Autodesk Fusion 360 part; units mm, degrees
(part 3 of 11)
  spline S34 degree 5 poles (-69.3976, -46.666) (-69.4262, -46.6856) (-69.4827, -46.7255) (-69.566, -46.7874) (-69.6741, -46.8736) (-69.8053, -46.9865) (-69.9336, -47.103) (-70.0602, -47.2219) (-70.1858, -47.342) (-70.3108, -47.4628) (-70.435, -47.5846) (-70.5583, -47.7074) (-70.6804, -47.8317) (-70.801, -47.9578) (-70.9202, -48.0856) (-71.038, -48.215) (-71.1547, -48.3457) (-71.2704, -48.4776) (-71.3852, -48.6104) (-71.4992, -48.7441) (-71.6124, -48.8787) (-71.7247, -49.0142) (-71.8361, -49.1508) (-71.9465, -49.2883) (-72.0561, -49.4269) (-72.1647, -49.5664) (-72.2724, -49.7069) (-72.3794, -49.8482) (-72.4855, -49.9903) (-72.5909, -50.1332) (-72.6954, -50.2769) (-72.7992, -50.4214) (-72.9023, -50.5667) (-73.0045, -50.7127) (-73.106, -50.8595) (-73.2067, -51.0071) (-73.3066, -51.1554) (-73.4058, -51.3044) (-73.5043, -51.4541) (-73.6021, -51.6045) (-73.6991, -51.7555) (-73.7954, -51.9073) (-73.8911, -52.0596) (-73.986, -52.2127) (-74.0802, -52.3664) (-74.1737, -52.5207) (-74.2665, -52.6757) (-74.3586, -52.8312) (-74.45, -52.9874) (-74.5408, -53.1442) (-74.6309, -53.3016) (-74.7203, -53.4595) (-74.8091, -53.618) (-74.8972, -53.7772) (-74.9846, -53.9368) (-75.0713, -54.097) (-75.1575, -54.2578) (-75.2429, -54.4191) (-75.3277, -54.581) (-75.4119, -54.7434) (-75.4954, -54.9063) (-75.5783, -55.0698) (-75.6605, -55.2337) (-75.7421, -55.3982) (-75.8231, -55.5632) (-75.9034, -55.7287) (-75.9831, -55.8946) (-76.0622, -56.0611) (-76.1407, -56.228) (-76.2185, -56.3954) (-76.2957, -56.5633) (-76.357, -56.698) (-76.4027, -56.7993) (-76.433, -56.8669) (-76.4482, -56.9007) knots 0 0 0 0 0 0 0.01428571 0.02857143 0.04285714 0.05714286 0.07142857 0.08571429 0.1 0.11428571 0.12857143 0.14285714 0.15714286 0.17142857 0.18571429 0.2 0.21428571 0.22857143 0.24285714 0.25714286 0.27142857 0.28571429 0.3 0.31428571 0.32857143 0.34285714 0.35714286 0.37142857 0.38571429 0.4 0.41428571 0.42857143 0.44285714 0.45714286 0.47142857 0.48571429 0.5 0.51428571 0.52857143 0.54285714 0.55714286 0.57142857 0.58571429 0.6 0.61428571 0.62857143 0.64285714 0.65714286 0.67142857 0.68571429 0.7 0.71428571 0.72857143 0.74285714 0.75714286 0.77142857 0.78571429 0.8 0.81428571 0.82857143 0.84285714 0.85714286 0.87142857 0.88571429 0.9 0.91428571 0.92857143 0.94285714 0.95714286 0.97142857 0.98571429 1 1 1 1 1 1
  arc A70 (-76.4482, -56.9007) -> (-73.5542, -60.5296) centre (-0.5538, 0.6546) ccw
  spline S35 degree 5 poles (-73.5542, -60.5296) (-73.5179, -60.5224) (-73.4452, -60.5078) (-73.3364, -60.4858) (-73.1914, -60.4561) (-73.0105, -60.4181) (-72.83, -60.3795) (-72.6498, -60.3402) (-72.4699, -60.3001) (-72.2904, -60.2593) (-72.1112, -60.2178) (-71.9323, -60.1756) (-71.7538, -60.1326) (-71.5756, -60.0889) (-71.3978, -60.0445) (-71.2204, -59.9993) (-71.0434, -59.9534) (-70.8667, -59.9067) (-70.6904, -59.8593) (-70.5145, -59.8112) (-70.339, -59.7622) (-70.1639, -59.7125) (-69.9891, -59.662) (-69.8148, -59.6108) (-69.6409, -59.5588) (-69.4675, -59.506) (-69.2944, -59.4524) (-69.1218, -59.398) (-68.9497, -59.3428) (-68.7779, -59.2868) (-68.6067, -59.2299) (-68.4359, -59.1723) (-68.2655, -59.1138) (-68.0957, -59.0545) (-67.9263, -58.9944) (-67.7575, -58.9334) (-67.5891, -58.8715) (-67.4212, -58.8088) (-67.2539, -58.7453) (-67.0871, -58.6808) (-66.9208, -58.6155) (-66.7551, -58.5492) (-66.5899, -58.4821) (-66.4254, -58.4139) (-66.2614, -58.3449) (-66.0981, -58.2749) (-65.9353, -58.204) (-65.7731, -58.1321) (-65.6116, -58.0593) (-65.4507, -57.9855) (-65.2905, -57.9107) (-65.131, -57.8347) (-64.9723, -57.7577) (-64.8144, -57.6795) (-64.6573, -57.6001) (-64.5009, -57.5197) (-64.3452, -57.4383) (-64.1901, -57.3559) (-64.0358, -57.2725) (-63.8824, -57.1878) (-63.7301, -57.1018) (-63.579, -57.014) (-63.4292, -56.9245) (-63.2808, -56.8331) (-63.1336, -56.7402) (-62.9873, -56.6462) (-62.8416, -56.5513) (-62.6966, -56.4555) (-62.5526, -56.3586) (-62.4104, -56.2594) (-62.2711, -56.1566) (-62.163, -56.0704) (-62.0842, -56.003) (-62.0327, -55.9567) (-62.0072, -55.9332) knots -1 -1 -1 -1 -1 -1 -0.98571429 -0.97142857 -0.95714286 -0.94285714 -0.92857143 -0.91428571 -0.9 -0.88571429 -0.87142857 -0.85714286 -0.84285714 -0.82857143 -0.81428571 -0.8 -0.78571429 -0.77142857 -0.75714286 -0.74285714 -0.72857143 -0.71428571 -0.7 -0.68571429 -0.67142857 -0.65714286 -0.64285714 -0.62857143 -0.61428571 -0.6 -0.58571429 -0.57142857 -0.55714286 -0.54285714 -0.52857143 -0.51428571 -0.5 -0.48571429 -0.47142857 -0.45714286 -0.44285714 -0.42857143 -0.41428571 -0.4 -0.38571429 -0.37142857 -0.35714286 -0.34285714 -0.32857143 -0.31428571 -0.3 -0.28571429 -0.27142857 -0.25714286 -0.24285714 -0.22857143 -0.21428571 -0.2 -0.18571429 -0.17142857 -0.15714286 -0.14285714 -0.12857143 -0.11428571 -0.1 -0.08571429 -0.07142857 -0.05714286 -0.04285714 -0.02857143 -0.01428571 0 0 0 0 0 0
  line L35 (-62.0072, -55.9332) -> (-60.9079, -54.9212)
  arc A71 (-59.7916, -54.9619) -> (-60.9079, -54.9212) centre (-60.3703, -55.5052) ccw
  arc A72 (-59.7916, -54.9619) -> (-56.1704, -58.5831) centre (-0.5538, 0.6546) ccw
  arc A73 (-56.1297, -59.6994) -> (-56.1704, -58.5831) centre (-56.7137, -59.1618) ccw
  line L36 (-56.1297, -59.6994) -> (-57.1417, -60.7988)
  spline S36 degree 5 poles (-57.1417, -60.7988) (-57.1652, -60.8242) (-57.2114, -60.8757) (-57.2789, -60.9545) (-57.3651, -61.0626) (-57.4679, -61.2019) (-57.5671, -61.3441) (-57.664, -61.4881) (-57.7597, -61.6331) (-57.8547, -61.7788) (-57.9487, -61.9251) (-58.0416, -62.0723) (-58.1329, -62.2207) (-58.2225, -62.3705) (-58.3102, -62.5216) (-58.3963, -62.6739) (-58.481, -62.8274) (-58.5644, -62.9817) (-58.6468, -63.1367) (-58.7282, -63.2924) (-58.8086, -63.4488) (-58.8879, -63.6059) (-58.9662, -63.7638) (-59.0432, -63.9225) (-59.1192, -64.082) (-59.194, -64.2422) (-59.2678, -64.4031) (-59.3406, -64.5647) (-59.4125, -64.7268) (-59.4834, -64.8896) (-59.5534, -65.053) (-59.6224, -65.2169) (-59.6905, -65.3815) (-59.7577, -65.5466) (-59.824, -65.7123) (-59.8893, -65.8786) (-59.9537, -66.0454) (-60.0173, -66.2127) (-60.08, -66.3806) (-60.1419, -66.549) (-60.2029, -66.7178) (-60.263, -66.8872) (-60.3223, -67.0571) (-60.3808, -67.2274) (-60.4384, -67.3982) (-60.4952, -67.5695) (-60.5512, -67.7412) (-60.6064, -67.9133) (-60.6608, -68.086) (-60.7144, -68.259) (-60.7673, -68.4325) (-60.8193, -68.6064) (-60.8705, -68.7807) (-60.921, -68.9554) (-60.9707, -69.1305) (-61.0196, -69.306) (-61.0678, -69.4819) (-61.1152, -69.6582) (-61.1619, -69.8349) (-61.2078, -70.0119) (-61.253, -70.1894) (-61.2974, -70.3672) (-61.3411, -70.5453) (-61.3841, -70.7238) (-61.4263, -70.9027) (-61.4678, -71.0819) (-61.5086, -71.2614) (-61.5486, -71.4413) (-61.588, -71.6215) (-61.6266, -71.8021) (-61.6645, -71.9829) (-61.6943, -72.1279) (-61.7163, -72.2367) (-61.7308, -72.3094) (-61.7381, -72.3457) knots 0 0 0 0 0 0 0.01428571 0.02857143 0.04285714 0.05714286 0.07142857 0.08571429 0.1 0.11428571 0.12857143 0.14285714 0.15714286 0.17142857 0.18571429 0.2 0.21428571 0.22857143 0.24285714 0.25714286 0.27142857 0.28571429 0.3 0.31428571 0.32857143 0.34285714 0.35714286 0.37142857 0.38571429 0.4 0.41428571 0.42857143 0.44285714 0.45714286 0.47142857 0.48571429 0.5 0.51428571 0.52857143 0.54285714 0.55714286 0.57142857 0.58571429 0.6 0.61428571 0.62857143 0.64285714 0.65714286 0.67142857 0.68571429 0.7 0.71428571 0.72857143 0.74285714 0.75714286 0.77142857 0.78571429 0.8 0.81428571 0.82857143 0.84285714 0.85714286 0.87142857 0.88571429 0.9 0.91428571 0.92857143 0.94285714 0.95714286 0.97142857 0.98571429 1 1 1 1 1 1
  arc A74 (-61.7381, -72.3457) -> (-58.1092, -75.2397) centre (-0.5538, 0.6546) ccw
  spline S37 degree 5 poles (-58.1092, -75.2397) (-58.0753, -75.2245) (-58.0078, -75.1942) (-57.9065, -75.1485) (-57.7718, -75.0873) (-57.6039, -75.01) (-57.4365, -74.9322) (-57.2696, -74.8537) (-57.1031, -74.7747) (-56.9371, -74.695) (-56.7717, -74.6146) (-56.6067, -74.5336) (-56.4422, -74.452) (-56.2783, -74.3698) (-56.1148, -74.2869) (-55.9519, -74.2034) (-55.7895, -74.1192) (-55.6276, -74.0344) (-55.4663, -73.949) (-55.3055, -73.8629) (-55.1453, -73.7761) (-54.9856, -73.6887) (-54.8265, -73.6006) (-54.668, -73.5118) (-54.51, -73.4224) (-54.3527, -73.3323) (-54.1959, -73.2416) (-54.0397, -73.1501) (-53.8842, -73.058) (-53.7292, -72.9652) (-53.5749, -72.8717) (-53.4212, -72.7775) (-53.2681, -72.6826) (-53.1157, -72.587) (-52.964, -72.4906) (-52.8129, -72.3936) (-52.6626, -72.2958) (-52.5129, -72.1974) (-52.3638, -72.0981) (-52.2156, -71.9982) (-52.068, -71.8975) (-51.9212, -71.796) (-51.7751, -71.6938) (-51.6299, -71.5908) (-51.4854, -71.487) (-51.3417, -71.3824) (-51.1988, -71.277) (-51.0567, -71.1709) (-50.9154, -71.0639) (-50.7749, -70.9562) (-50.6354, -70.8476) (-50.4968, -70.7381) (-50.3592, -70.6276) (-50.2227, -70.5162) (-50.0871, -70.4039) (-49.9526, -70.2907) (-49.8189, -70.1767) (-49.6861, -70.0619) (-49.5542, -69.9462) (-49.4235, -69.8295) (-49.2941, -69.7117) (-49.1663, -69.5925) (-49.0402, -69.4719) (-48.9159, -69.3498) (-48.793, -69.2265) (-48.6713, -69.1023) (-48.5504, -68.9773) (-48.4304, -68.8517) (-48.3115, -68.7252) (-48.1949, -68.5968) (-48.082, -68.4657) (-47.9958, -68.3575) (-47.934, -68.2742) (-47.8941, -68.2177) (-47.8745, -68.1891) knots -1 -1 -1 -1 -1 -1 -0.98571429 -0.97142857 -0.95714286 -0.94285714 -0.92857143 -0.91428571 -0.9 -0.88571429 -0.87142857 -0.85714286 -0.84285714 -0.82857143 -0.81428571 -0.8 -0.78571429 -0.77142857 -0.75714286 -0.74285714 -0.72857143 -0.71428571 -0.7 -0.68571429 -0.67142857 -0.65714286 -0.64285714 -0.62857143 -0.61428571 -0.6 -0.58571429 -0.57142857 -0.55714286 -0.54285714 -0.52857143 -0.51428571 -0.5 -0.48571429 -0.47142857 -0.45714286 -0.44285714 -0.42857143 -0.41428571 -0.4 -0.38571429 -0.37142857 -0.35714286 -0.34285714 -0.32857143 -0.31428571 -0.3 -0.28571429 -0.27142857 -0.25714286 -0.24285714 -0.22857143 -0.21428571 -0.2 -0.18571429 -0.17142857 -0.15714286 -0.14285714 -0.12857143 -0.11428571 -0.1 -0.08571429 -0.07142857 -0.05714286 -0.04285714 -0.02857143 -0.01428571 0 0 0 0 0 0
  line L37 (-47.8745, -68.1891) -> (-47.0279, -66.9578)
  arc A75 (-45.9305, -66.7491) -> (-47.0279, -66.9578) centre (-46.3738, -67.4076) ccw
  arc A76 (-45.9305, -66.7491) -> (-41.5943, -69.4737) centre (-0.5538, 0.6546) ccw
  arc A77 (-41.3063, -70.553) -> (-41.5943, -69.4737) centre (-41.9952, -70.1588) ccw
  line L38 (-41.3063, -70.553) -> (-42.0483, -71.85)
  spline S38 degree 5 poles (-42.0483, -71.85) (-42.0655, -71.88) (-42.0991, -71.9405) (-42.1473, -72.0324) (-42.2074, -72.157) (-42.2766, -72.3156) (-42.3416, -72.4763) (-42.4041, -72.6383) (-42.4651, -72.801) (-42.5253, -72.9641) (-42.5844, -73.1277) (-42.6422, -73.2919) (-42.6982, -73.4569) (-42.7522, -73.6228) (-42.8041, -73.7896) (-42.8542, -73.9573) (-42.9025, -74.1257) (-42.9496, -74.2947) (-42.9954, -74.4642) (-43.0401, -74.6341) (-43.0837, -74.8045) (-43.1261, -74.9753) (-43.1672, -75.1467) (-43.207, -75.3185) (-43.2456, -75.4909) (-43.2829, -75.6638) (-43.319, -75.8371) (-43.354, -76.0108) (-43.388, -76.1848) (-43.4209, -76.3593) (-43.4528, -76.5342) (-43.4836, -76.7094) (-43.5134, -76.885) (-43.5422, -77.0609) (-43.5699, -77.2372) (-43.5966, -77.4138) (-43.6223, -77.5908) (-43.6471, -77.7681) (-43.6708, -77.9457) (-43.6937, -78.1236) (-43.7155, -78.3018) (-43.7365, -78.4803) (-43.7565, -78.6591) (-43.7756, -78.8382) (-43.7938, -79.0175) (-43.8111, -79.1971) (-43.8275, -79.377) (-43.843, -79.5572) (-43.8576, -79.7375) (-43.8714, -79.9182) (-43.8842, -80.0991) (-43.8963, -80.2802) (-43.9075, -80.4615) (-43.9178, -80.6431) (-43.9273, -80.8249) (-43.9359, -81.0069) (-43.9437, -81.1891) (-43.9507, -81.3715) (-43.9569, -81.5541) (-43.9623, -81.737) (-43.9669, -81.92) (-43.9706, -82.1032) (-43.9736, -82.2866) (-43.9757, -82.4702) (-43.9771, -82.654) (-43.9777, -82.8379) (-43.9775, -83.022) (-43.9765, -83.2063) (-43.9748, -83.3908) (-43.9723, -83.5754) (-43.969, -83.7602) (-43.9657, -83.9081) (-43.963, -84.0191) (-43.961, -84.0932) (-43.9599, -84.1302) knots 0 0 0 0 0 0 0.01428571 0.02857143 0.04285714 0.05714286 0.07142857 0.08571429 0.1 0.11428571 0.12857143 0.14285714 0.15714286 0.17142857 0.18571429 0.2 0.21428571 0.22857143 0.24285714 0.25714286 0.27142857 0.28571429 0.3 0.31428571 0.32857143 0.34285714 0.35714286 0.37142857 0.38571429 0.4 0.41428571 0.42857143 0.44285714 0.45714286 0.47142857 0.48571429 0.5 0.51428571 0.52857143 0.54285714 0.55714286 0.57142857 0.58571429 0.6 0.61428571 0.62857143 0.64285714 0.65714286 0.67142857 0.68571429 0.7 0.71428571 0.72857143 0.74285714 0.75714286 0.77142857 0.78571429 0.8 0.81428571 0.82857143 0.84285714 0.85714286 0.87142857 0.88571429 0.9 0.91428571 0.92857143 0.94285714 0.95714286 0.97142857 0.98571429 1 1 1 1 1 1
  arc A78 (-43.9599, -84.1302) -> (-39.7781, -86.1441) centre (-0.5538, 0.6546) ccw
  spline S39 degree 5 poles (-39.7781, -86.1441) (-39.7485, -86.1218) (-39.6893, -86.0772) (-39.6008, -86.0102) (-39.4831, -85.9205) (-39.3366, -85.8078) (-39.1907, -85.6947) (-39.0454, -85.581) (-38.9007, -85.4669) (-38.7566, -85.3522) (-38.6132, -85.2371) (-38.4704, -85.1214) (-38.3282, -85.0053) (-38.1866, -84.8886) (-38.0457, -84.7715) (-37.9055, -84.6538) (-37.7659, -84.5356) (-37.6269, -84.4169) (-37.4887, -84.2977) (-37.3511, -84.178) (-37.2142, -84.0577) (-37.078, -83.9369) (-36.9425, -83.8157) (-36.8076, -83.6939) (-36.6735, -83.5715) (-36.5402, -83.4487) (-36.4075, -83.3253) (-36.2756, -83.2014) (-36.1444, -83.077) (-36.014, -82.952) (-35.8844, -82.8265) (-35.7555, -82.7005) (-35.6274, -82.5739) (-35.5001, -82.4468) (-35.3736, -82.3191) (-35.2479, -82.1909) (-35.1231, -82.0621) (-34.999, -81.9328) (-34.8758, -81.8029) (-34.7535, -81.6724) (-34.6321, -81.5414) (-34.5115, -81.4098) (-34.3919, -81.2777) (-34.2732, -81.1449) (-34.1554, -81.0116) (-34.0386, -80.8776) (-33.9227, -80.7431) (-33.8078, -80.608) (-33.6938, -80.4723) (-33.5809, -80.336) (-33.469, -80.1991) (-33.3583, -80.0615) (-33.2487, -79.9232) (-33.1404, -79.7842) (-33.0332, -79.6445) (-32.9272, -79.5042) (-32.8222, -79.3633) (-32.7183, -79.2218) (-32.6155, -79.0797) (-32.514, -78.9369) (-32.4141, -78.7932) (-32.316, -78.6486) (-32.2199, -78.5029) (-32.1259, -78.3563) (-32.0336, -78.2087) (-31.9425, -78.0605) (-31.8525, -77.9118) (-31.7634, -77.7626) (-31.6757, -77.6127) (-31.5906, -77.4617) (-31.5097, -77.3087) (-31.4497, -77.1841) (-31.408, -77.0891) (-31.3817, -77.0251) (-31.3689, -76.9929) knots -1 -1 -1 -1 -1 -1 -0.98571429 -0.97142857 -0.95714286 -0.94285714 -0.92857143 -0.91428571 -0.9 -0.88571429 -0.87142857 -0.85714286 -0.84285714 -0.82857143 -0.81428571 -0.8 -0.78571429 -0.77142857 -0.75714286 -0.74285714 -0.72857143 -0.71428571 -0.7 -0.68571429 -0.67142857 -0.65714286 -0.64285714 -0.62857143 -0.61428571 -0.6 -0.58571429 -0.57142857 -0.55714286 -0.54285714 -0.52857143 -0.51428571 -0.5 -0.48571429 -0.47142857 -0.45714286 -0.44285714 -0.42857143 -0.41428571 -0.4 -0.38571429 -0.37142857 -0.35714286 -0.34285714 -0.32857143 -0.31428571 -0.3 -0.28571429 -0.27142857 -0.25714286 -0.24285714 -0.22857143 -0.21428571 -0.2 -0.18571429 -0.17142857 -0.15714286 -0.14285714 -0.12857143 -0.11428571 -0.1 -0.08571429 -0.07142857 -0.05714286 -0.04285714 -0.02857143 -0.01428571 0 0 0 0 0 0
  line L39 (-31.3689, -76.9929) -> (-30.8175, -75.6041)
  arc A79 (-29.7941, -75.1564) -> (-30.8175, -75.6041) centre (-30.0797, -75.897) ccw
  arc A80 (-29.7941, -75.1564) -> (-24.9603, -76.8478) centre (-0.5538, 0.6546) ccw
  arc A81 (-24.4393, -77.8359) -> (-24.9603, -76.8478) centre (-25.1987, -77.6049) ccw
  line L40 (-24.4393, -77.8359) -> (-24.8741, -79.2655)
  spline S40 degree 5 poles (-24.8741, -79.2655) (-24.8842, -79.2987) (-24.9035, -79.3651) (-24.9301, -79.4654) (-24.9609, -79.6002) (-24.9931, -79.7703) (-25.0207, -79.9414) (-25.0456, -80.1132) (-25.0689, -80.2854) (-25.0912, -80.4578) (-25.1125, -80.6305) (-25.1323, -80.8034) (-25.1502, -80.9767) (-25.1659, -81.1505) (-25.1794, -81.3247) (-25.1909, -81.4994) (-25.2006, -81.6743) (-25.2088, -81.8495) (-25.2158, -82.0249) (-25.2216, -82.2005) (-25.2261, -82.3763) (-25.2294, -82.5523) (-25.2314, -82.7285) (-25.232, -82.905) (-25.2312, -83.0816) (-25.2291, -83.2584) (-25.2258, -83.4354) (-25.2213, -83.6125) (-25.2157, -83.7898) (-25.209, -83.9672) (-25.2011, -84.1448) (-25.1922, -84.3225) (-25.1822, -84.5003) (-25.171, -84.6782) (-25.1588, -84.8563) (-25.1456, -85.0344) (-25.1312, -85.2127) (-25.1159, -85.391) (-25.0996, -85.5695) (-25.0822, -85.748) (-25.0639, -85.9266) (-25.0446, -86.1053) (-25.0244, -86.2841) (-25.0031, -86.4629) (-24.981, -86.6418) (-24.9578, -86.8207) (-24.9338, -86.9998) (-24.9088, -87.1788) (-24.8829, -87.3579) (-24.8562, -87.5371) (-24.8285, -87.7163) (-24.7999, -87.8956) (-24.7705, -88.0748) (-24.7401, -88.2541) (-24.7089, -88.4335) (-24.6769, -88.6129) (-24.6439, -88.7922) (-24.6102, -88.9717) (-24.5755, -89.1511) (-24.5401, -89.3305) (-24.5038, -89.51) (-24.4667, -89.6894) (-24.4288, -89.8689) (-24.39, -90.0484) (-24.3505, -90.2278) (-24.3101, -90.4073) (-24.2689, -90.5868) (-24.227, -90.7662) (-24.1843, -90.9456) (-24.1407, -91.1251) (-24.0964, -91.3045) (-24.0603, -91.448) (-24.0329, -91.5556) (-24.0145, -91.6274) (-24.0053, -91.6633) knots 0 0 0 0 0 0 0.01428571 0.02857143 0.04285714 0.05714286 0.07142857 0.08571429 0.1 0.11428571 0.12857143 0.14285714 0.15714286 0.17142857 0.18571429 0.2 0.21428571 0.22857143 0.24285714 0.25714286 0.27142857 0.28571429 0.3 0.31428571 0.32857143 0.34285714 0.35714286 0.37142857 0.38571429 0.4 0.41428571 0.42857143 0.44285714 0.45714286 0.47142857 0.48571429 0.5 0.51428571 0.52857143 0.54285714 0.55714286 0.57142857 0.58571429 0.6 0.61428571 0.62857143 0.64285714 0.65714286 0.67142857 0.68571429 0.7 0.71428571 0.72857143 0.74285714 0.75714286 0.77142857 0.78571429 0.8 0.81428571 0.82857143 0.84285714 0.85714286 0.87142857 0.88571429 0.9 0.91428571 0.92857143 0.94285714 0.95714286 0.97142857 0.98571429 1 1 1 1 1 1
  arc A82 (-24.0053, -91.6633) -> (-19.4801, -92.6961) centre (-0.5538, 0.6546) ccw
  spline S41 degree 5 poles (-19.4801, -92.6961) (-19.4562, -92.6678) (-19.4084, -92.6111) (-19.3371, -92.5261) (-19.2423, -92.4124) (-19.1245, -92.27) (-19.0075, -92.1272) (-18.8911, -91.9841) (-18.7754, -91.8406) (-18.6605, -91.6968) (-18.5462, -91.5526) (-18.4327, -91.4081) (-18.32, -91.2632) (-18.2079, -91.118) (-18.0966, -90.9724) (-17.9861, -90.8264) (-17.8763, -90.6801) (-17.7672, -90.5335) (-17.659, -90.3865) (-17.5515, -90.2392) (-17.4448, -90.0915) (-17.3388, -89.9434) (-17.2337, -89.795) (-17.1294, -89.6463) (-17.0259, -89.4972) (-16.9232, -89.3478) (-16.8213, -89.198) (-16.7203, -89.0478) (-16.6201, -88.8973) (-16.5207, -88.7465) (-16.4223, -88.5953) (-16.3247, -88.4437) (-16.2279, -88.2918) (-16.1321, -88.1395) (-16.0372, -87.9869) (-15.9432, -87.8339) (-15.8501, -87.6806) (-15.758, -87.5269) (-15.6668, -87.3729) (-15.5766, -87.2185) (-15.4873, -87.0637) (-15.399, -86.9086) (-15.3118, -86.7531) (-15.2256, -86.5973) (-15.1405, -86.4411) (-15.0564, -86.2845) (-14.9734, -86.1276) (-14.8914, -85.9703) (-14.8105, -85.8126) (-14.7307, -85.6546) (-14.6521, -85.4962) (-14.5748, -85.3374) (-14.4987, -85.1782) (-14.424, -85.0186) (-14.3507, -84.8586) (-14.2785, -84.6982) (-14.2075, -84.5375) (-14.1377, -84.3764) (-14.0691, -84.215) (-14.0019, -84.0532) (-13.9365, -83.8909) (-13.873, -83.728) (-13.8118, -83.5647) (-13.7527, -83.4007) (-13.6955, -83.2363) (-13.6398, -83.0716) (-13.5851, -82.9065) (-13.5314, -82.7413) (-13.4793, -82.5757) (-13.4299, -82.4095) (-13.3851, -82.2423) (-13.3544, -82.1075) (-13.3348, -82.0056) (-13.3234, -81.9373) (-13.3181, -81.9031) knots -1 -1 -1 -1 -1 -1 -0.98571429 -0.97142857 -0.95714286 -0.94285714 -0.92857143 -0.91428571 -0.9 -0.88571429 -0.87142857 -0.85714286 -0.84285714 -0.82857143 -0.81428571 -0.8 -0.78571429 -0.77142857 -0.75714286 -0.74285714 -0.72857143 -0.71428571 -0.7 -0.68571429 -0.67142857 -0.65714286 -0.64285714 -0.62857143 -0.61428571 -0.6 -0.58571429 -0.57142857 -0.55714286 -0.54285714 -0.52857143 -0.51428571 -0.5 -0.48571429 -0.47142857 -0.45714286 -0.44285714 -0.42857143 -0.41428571 -0.4 -0.38571429 -0.37142857 -0.35714286 -0.34285714 -0.32857143 -0.31428571 -0.3 -0.28571429 -0.27142857 -0.25714286 -0.24285714 -0.22857143 -0.21428571 -0.2 -0.18571429 -0.17142857 -0.15714286 -0.14285714 -0.12857143 -0.11428571 -0.1 -0.08571429 -0.07142857 -0.05714286 -0.04285714 -0.02857143 -0.01428571 0 0 0 0 0 0
  line L41 (-13.3181, -81.9031) -> (-13.0895, -80.4264)
  arc A83 (-12.1914, -79.7623) -> (-13.0895, -80.4264) centre (-12.3051, -80.5478) ccw
  arc A84 (-12.1914, -79.7623) -> (-7.1025, -80.3356) centre (-0.5538, 0.6546) ccw
  arc A85 (-6.3747, -81.183) -> (-7.1025, -80.3356) centre (-7.1664, -81.1268) ccw
  line L42 (-6.3747, -81.183) -> (-6.4805, -82.6735)
  spline S42 degree 5 poles (-6.4805, -82.6735) (-6.4829, -82.7081) (-6.487, -82.7772) (-6.4906, -82.8808) (-6.4906, -83.0191) (-6.4841, -83.1921) (-6.473, -83.3651) (-6.459, -83.5381) (-6.4434, -83.7112) (-6.4268, -83.8843) (-6.4091, -84.0573) (-6.39, -84.2303) (-6.3689, -84.4033) (-6.3455, -84.5762) (-6.3199, -84.749) (-6.2922, -84.9218) (-6.2627, -85.0946) (-6.2318, -85.2672) (-6.1995, -85.4398) (-6.1661, -85.6123) (-6.1314, -85.7847) (-6.0955, -85.957) (-6.0582, -86.1292) (-6.0195, -86.3013) (-5.9794, -86.4734) (-5.9381, -86.6453) (-5.8954, -86.8171) (-5.8516, -86.9888) (-5.8067, -87.1604) (-5.7607, -87.3319) (-5.7135, -87.5032) (-5.6653, -87.6745) (-5.6159, -87.8456) (-5.5655, -88.0166) (-5.514, -88.1874) (-5.4614, -88.3582) (-5.4078, -88.5288) (-5.3531, -88.6993) (-5.2975, -88.8696) (-5.2409, -89.0398) (-5.1833, -89.2098) (-5.1247, -89.3798) (-5.0652, -89.5495) (-5.0047, -89.7191) (-4.9432, -89.8886) (-4.8809, -90.058) (-4.8176, -90.2271) (-4.7534, -90.3962) (-4.6883, -90.565) (-4.6223, -90.7337) (-4.5555, -90.9023) (-4.4877, -91.0707) (-4.4191, -91.2389) (-4.3497, -91.407) (-4.2793, -91.5749) (-4.2082, -91.7426) (-4.1361, -91.9102) (-4.0633, -92.0776) (-3.9896, -92.2448) (-3.9151, -92.4119) (-3.8398, -92.5787) (-3.7637, -92.7454) (-3.6868, -92.912) (-3.6091, -93.0783) (-3.5306, -93.2445) (-3.4513, -93.4105) (-3.3712, -93.5763) (-3.2904, -93.7419) (-3.2088, -93.9073) (-3.1264, -94.0725) (-3.0433, -94.2376) (-2.9762, -94.3695) (-2.9255, -94.4683) (-2.8916, -94.5342) (-2.8746, -94.5671) knots 0 0 0 0 0 0 0.01428571 0.02857143 0.04285714 0.05714286 0.07142857 0.08571429 0.1 0.11428571 0.12857143 0.14285714 0.15714286 0.17142857 0.18571429 0.2 0.21428571 0.22857143 0.24285714 0.25714286 0.27142857 0.28571429 0.3 0.31428571 0.32857143 0.34285714 0.35714286 0.37142857 0.38571429 0.4 0.41428571 0.42857143 0.44285714 0.45714286 0.47142857 0.48571429 0.5 0.51428571 0.52857143 0.54285714 0.55714286 0.57142857 0.58571429 0.6 0.61428571 0.62857143 0.64285714 0.65714286 0.67142857 0.68571429 0.7 0.71428571 0.72857143 0.74285714 0.75714286 0.77142857 0.78571429 0.8 0.81428571 0.82857143 0.84285714 0.85714286 0.87142857 0.88571429 0.9 0.91428571 0.92857143 0.94285714 0.95714286 0.97142857 0.98571429 1 1 1 1 1 1
  arc A86 (-2.8746, -94.5671) -> (1.7669, -94.5671) centre (-0.5538, 0.6546) ccw
  spline S43 degree 5 poles (1.7669, -94.5671) (1.7839, -94.5342) (1.8179, -94.4683) (1.8685, -94.3695) (1.9356, -94.2376) (2.0188, -94.0725) (2.1011, -93.9073) (2.1827, -93.7419) (2.2636, -93.5763) (2.3436, -93.4105) (2.4229, -93.2445) (2.5014, -93.0783) (2.5791, -92.912) (2.656, -92.7454) (2.7321, -92.5787) (2.8074, -92.4119) (2.8819, -92.2448) (2.9556, -92.0776) (3.0285, -91.9102) (3.1005, -91.7426) (3.1716, -91.5749) (3.242, -91.407) (3.3114, -91.2389) (3.3801, -91.0707) (3.4478, -90.9023) (3.5147, -90.7337) (3.5806, -90.565) (3.6457, -90.3962) (3.7099, -90.2271) (3.7732, -90.058) (3.8356, -89.8886) (3.897, -89.7191) (3.9575, -89.5495) (4.017, -89.3798) (4.0756, -89.2098) (4.1332, -89.0398) (4.1898, -88.8696) (4.2454, -88.6993) (4.3001, -88.5288) (4.3537, -88.3582) (4.4063, -88.1874) (4.4578, -88.0166) (4.5082, -87.8456) (4.5576, -87.6745) (4.6058, -87.5032) (4.653, -87.3319) (4.699, -87.1604) (4.7439, -86.9888) (4.7877, -86.8171) (4.8304, -86.6453) (4.8717, -86.4734) (4.9118, -86.3013) (4.9505, -86.1292) (4.9878, -85.957) (5.0237, -85.7847) (5.0584, -85.6123) (5.0918, -85.4398) (5.1241, -85.2672) (5.155, -85.0946) (5.1845, -84.9218) (5.2122, -84.749) (5.2378, -84.5762) (5.2612, -84.4033) (5.2823, -84.2303) (5.3014, -84.0573) (5.3191, -83.8843) (5.3357, -83.7112) (5.3513, -83.5381) (5.3653, -83.3651) (5.3764, -83.1921) (5.3829, -83.0191) (5.3829, -82.8808) (5.3793, -82.7772) (5.3752, -82.7081) (5.3728, -82.6735) knots -1 -1 -1 -1 -1 -1 -0.98571429 -0.97142857 -0.95714286 -0.94285714 -0.92857143 -0.91428571 -0.9 -0.88571429 -0.87142857 -0.85714286 -0.84285714 -0.82857143 -0.81428571 -0.8 -0.78571429 -0.77142857 -0.75714286 -0.74285714 -0.72857143 -0.71428571 -0.7 -0.68571429 -0.67142857 -0.65714286 -0.64285714 -0.62857143 -0.61428571 -0.6 -0.58571429 -0.57142857 -0.55714286 -0.54285714 -0.52857143 -0.51428571 -0.5 -0.48571429 -0.47142857 -0.45714286 -0.44285714 -0.42857143 -0.41428571 -0.4 -0.38571429 -0.37142857 -0.35714286 -0.34285714 -0.32857143 -0.31428571 -0.3 -0.28571429 -0.27142857 -0.25714286 -0.24285714 -0.22857143 -0.21428571 -0.2 -0.18571429 -0.17142857 -0.15714286 -0.14285714 -0.12857143 -0.11428571 -0.1 -0.08571429 -0.07142857 -0.05714286 -0.04285714 -0.02857143 -0.01428571 0 0 0 0 0 0
  line L43 (5.3728, -82.6735) -> (5.267, -81.183)
  arc A87 (5.9948, -80.3356) -> (5.267, -81.183) centre (6.0588, -81.1268) ccw
  arc A88 (5.9948, -80.3356) -> (11.0838, -79.7623) centre (-0.5538, 0.6546) ccw
  arc A89 (11.9819, -80.4264) -> (11.0838, -79.7623) centre (11.1974, -80.5478) ccw
  line L44 (11.9819, -80.4264) -> (12.2104, -81.9031)
  spline S44 degree 5 poles (12.2104, -81.9031) (12.2157, -81.9373) (12.2271, -82.0056) (12.2467, -82.1075) (12.2774, -82.2423) (12.3222, -82.4095) (12.3716, -82.5757) (12.4237, -82.7413) (12.4774, -82.9065) (12.5321, -83.0716) (12.5879, -83.2363) (12.645, -83.4007) (12.7041, -83.5647) (12.7654, -83.728) (12.8288, -83.8909) (12.8942, -84.0532) (12.9614, -84.215) (13.03, -84.3764) (13.0998, -84.5375) (13.1708, -84.6982) (13.243, -84.8586) (13.3164, -85.0186) (13.3911, -85.1782) (13.4671, -85.3374) (13.5444, -85.4962) (13.623, -85.6546) (13.7028, -85.8126) (13.7837, -85.9703) (13.8657, -86.1276) (13.9487, -86.2845) (14.0328, -86.4411) (14.118, -86.5973) (14.2041, -86.7531) (14.2914, -86.9086) (14.3796, -87.0637) (14.4689, -87.2185) (14.5591, -87.3729) (14.6503, -87.5269) (14.7425, -87.6806) (14.8355, -87.8339) (14.9295, -87.9869) (15.0244, -88.1395) (15.1203, -88.2918) (15.217, -88.4437) (15.3146, -88.5953) (15.4131, -88.7465) (15.5124, -88.8973) (15.6126, -89.0478) (15.7136, -89.198) (15.8155, -89.3478) (15.9182, -89.4972) (16.0217, -89.6463) (16.126, -89.795) (16.2312, -89.9434) (16.3371, -90.0915) (16.4438, -90.2392) (16.5513, -90.3865) (16.6596, -90.5335) (16.7686, -90.6801) (16.8784, -90.8264) (16.9889, -90.9724) (17.1002, -91.118) (17.2123, -91.2632) (17.3251, -91.4081) (17.4386, -91.5526) (17.5528, -91.6968) (17.6677, -91.8406) (17.7834, -91.9841) (17.8998, -92.1272) (18.0168, -92.27) (18.1346, -92.4124) (18.2294, -92.5261) (18.3008, -92.6111) (18.3485, -92.6678) (18.3724, -92.6961) knots 0 0 0 0 0 0 0.01428571 0.02857143 0.04285714 0.05714286 0.07142857 0.08571429 0.1 0.11428571 0.12857143 0.14285714 0.15714286 0.17142857 0.18571429 0.2 0.21428571 0.22857143 0.24285714 0.25714286 0.27142857 0.28571429 0.3 0.31428571 0.32857143 0.34285714 0.35714286 0.37142857 0.38571429 0.4 0.41428571 0.42857143 0.44285714 0.45714286 0.47142857 0.48571429 0.5 0.51428571 0.52857143 0.54285714 0.55714286 0.57142857 0.58571429 0.6 0.61428571 0.62857143 0.64285714 0.65714286 0.67142857 0.68571429 0.7 0.71428571 0.72857143 0.74285714 0.75714286 0.77142857 0.78571429 0.8 0.81428571 0.82857143 0.84285714 0.85714286 0.87142857 0.88571429 0.9 0.91428571 0.92857143 0.94285714 0.95714286 0.97142857 0.98571429 1 1 1 1 1 1
  arc A90 (18.3724, -92.6961) -> (22.8976, -91.6633) centre (-0.5538, 0.6546) ccw
  spline S45 degree 5 poles (22.8976, -91.6633) (22.9068, -91.6274) (22.9253, -91.5556) (22.9527, -91.448) (22.9887, -91.3045) (23.033, -91.1251) (23.0766, -90.9456) (23.1193, -90.7662) (23.1613, -90.5868) (23.2024, -90.4073) (23.2428, -90.2278) (23.2823, -90.0484) (23.3211, -89.8689) (23.359, -89.6894) (23.3961, -89.51) (23.4324, -89.3305) (23.4679, -89.1511) (23.5025, -88.9717) (23.5362, -88.7922) (23.5692, -88.6129) (23.6012, -88.4335) (23.6324, -88.2541) (23.6628, -88.0748) (23.6922, -87.8956) (23.7208, -87.7163) (23.7485, -87.5371) (23.7753, -87.3579) (23.8011, -87.1788) (23.8261, -86.9998) (23.8502, -86.8207) (23.8733, -86.6418) (23.8955, -86.4629) (23.9167, -86.2841) (23.9369, -86.1053) (23.9562, -85.9266) (23.9746, -85.748) (23.9919, -85.5695) (24.0082, -85.391) (24.0236, -85.2127) (24.0379, -85.0344) (24.0512, -84.8563) (24.0634, -84.6782) (24.0745, -84.5003) (24.0845, -84.3225) (24.0934, -84.1448) (24.1013, -83.9672) (24.108, -83.7898) (24.1136, -83.6125) (24.1181, -83.4354) (24.1214, -83.2584) (24.1235, -83.0816) (24.1243, -82.905) (24.1237, -82.7285) (24.1218, -82.5523) (24.1185, -82.3763) (24.1139, -82.2005) (24.1081, -82.0249) (24.1011, -81.8495) (24.0929, -81.6743) (24.0832, -81.4994) (24.0717, -81.3247) (24.0582, -81.1505) (24.0425, -80.9767) (24.0246, -80.8034) (24.0048, -80.6305) (23.9836, -80.4578) (23.9612, -80.2854) (23.9379, -80.1132) (23.913, -79.9414) (23.8854, -79.7703) (23.8532, -79.6002) (23.8224, -79.4654) (23.7959, -79.3651) (23.7765, -79.2987) (23.7664, -79.2655) knots -1 -1 -1 -1 -1 -1 -0.98571429 -0.97142857 -0.95714286 -0.94285714 -0.92857143 -0.91428571 -0.9 -0.88571429 -0.87142857 -0.85714286 -0.84285714 -0.82857143 -0.81428571 -0.8 -0.78571429 -0.77142857 -0.75714286 -0.74285714 -0.72857143 -0.71428571 -0.7 -0.68571429 -0.67142857 -0.65714286 -0.64285714 -0.62857143 -0.61428571 -0.6 -0.58571429 -0.57142857 -0.55714286 -0.54285714 -0.52857143 -0.51428571 -0.5 -0.48571429 -0.47142857 -0.45714286 -0.44285714 -0.42857143 -0.41428571 -0.4 -0.38571429 -0.37142857 -0.35714286 -0.34285714 -0.32857143 -0.31428571 -0.3 -0.28571429 -0.27142857 -0.25714286 -0.24285714 -0.22857143 -0.21428571 -0.2 -0.18571429 -0.17142857 -0.15714286 -0.14285714 -0.12857143 -0.11428571 -0.1 -0.08571429 -0.07142857 -0.05714286 -0.04285714 -0.02857143 -0.01428571 0 0 0 0 0 0
  line L45 (23.7664, -79.2655) -> (23.3316, -77.8359)
  arc A91 (23.8526, -76.8478) -> (23.3316, -77.8359) centre (24.091, -77.6049) ccw
  arc A92 (23.8526, -76.8478) -> (28.6864, -75.1564) centre (-0.5538, 0.6546) ccw
  arc A93 (29.7098, -75.6041) -> (28.6864, -75.1564) centre (28.9721, -75.897) ccw
  line L46 (29.7098, -75.6041) -> (30.2612, -76.9929)
  spline S46 degree 5 poles (30.2612, -76.9929) (30.274, -77.0251) (30.3003, -77.0891) (30.342, -77.1841) (30.402, -77.3087) (30.4829, -77.4617) (30.568, -77.6127) (30.6557, -77.7626) (30.7448, -77.9118) (30.8349, -78.0605) (30.9259, -78.2087) (31.0182, -78.3563) (31.1123, -78.5029) (31.2083, -78.6486) (31.3064, -78.7932) (31.4063, -78.9369) (31.5078, -79.0797) (31.6106, -79.2218) (31.7145, -79.3633) (31.8195, -79.5042) (31.9255, -79.6445) (32.0327, -79.7842) (32.141, -79.9232) (32.2506, -80.0615) (32.3613, -80.1991) (32.4732, -80.336) (32.5861, -80.4723) (32.7001, -80.608) (32.815, -80.7431) (32.9309, -80.8776) (33.0477, -81.0116) (33.1655, -81.1449) (33.2842, -81.2777) (33.4038, -81.4098) (33.5244, -81.5414) (33.6458, -81.6724) (33.7682, -81.8029) (33.8914, -81.9328) (34.0154, -82.0621) (34.1403, -82.1909) (34.2659, -82.3191) (34.3924, -82.4468) (34.5197, -82.5739) (34.6478, -82.7005) (34.7767, -82.8265) (34.9063, -82.952) (35.0368, -83.077) (35.1679, -83.2014) (35.2998, -83.3253) (35.4325, -83.4487) (35.5659, -83.5715) (35.7, -83.6939) (35.8348, -83.8157) (35.9703, -83.9369) (36.1065, -84.0577) (36.2434, -84.178) (36.381, -84.2977) (36.5193, -84.4169) (36.6582, -84.5356) (36.7978, -84.6538) (36.938, -84.7715) (37.0789, -84.8886) (37.2205, -85.0053) (37.3627, -85.1214) (37.5055, -85.2371) (37.649, -85.3522) (37.793, -85.4669) (37.9377, -85.581) (38.083, -85.6947) (38.2289, -85.8078) (38.3754, -85.9205) (38.4931, -86.0102) (38.5816, -86.0772) (38.6408, -86.1218) (38.6704, -86.1441) knots 0 0 0 0 0 0 0.01428571 0.02857143 0.04285714 0.05714286 0.07142857 0.08571429 0.1 0.11428571 0.12857143 0.14285714 0.15714286 0.17142857 0.18571429 0.2 0.21428571 0.22857143 0.24285714 0.25714286 0.27142857 0.28571429 0.3 0.31428571 0.32857143 0.34285714 0.35714286 0.37142857 0.38571429 0.4 0.41428571 0.42857143 0.44285714 0.45714286 0.47142857 0.48571429 0.5 0.51428571 0.52857143 0.54285714 0.55714286 0.57142857 0.58571429 0.6 0.61428571 0.62857143 0.64285714 0.65714286 0.67142857 0.68571429 0.7 0.71428571 0.72857143 0.74285714 0.75714286 0.77142857 0.78571429 0.8 0.81428571 0.82857143 0.84285714 0.85714286 0.87142857 0.88571429 0.9 0.91428571 0.92857143 0.94285714 0.95714286 0.97142857 0.98571429 1 1 1 1 1 1
  arc A94 (38.6704, -86.1441) -> (42.8523, -84.1302) centre (-0.5538, 0.6546) ccw
  spline S47 degree 5 poles (42.8523, -84.1302) (42.8533, -84.0932) (42.8553, -84.0191) (42.8581, -83.9081) (42.8613, -83.7602) (42.8646, -83.5754) (42.8671, -83.3908) (42.8688, -83.2063) (42.8698, -83.022) (42.87, -82.8379) (42.8694, -82.654) (42.868, -82.4702) (42.8659, -82.2866) (42.8629, -82.1032) (42.8592, -81.92) (42.8546, -81.737) (42.8492, -81.5541) (42.8431, -81.3715) (42.8361, -81.1891) (42.8282, -81.0069) (42.8196, -80.8249) (42.8101, -80.6431) (42.7998, -80.4615) (42.7886, -80.2802) (42.7766, -80.0991) (42.7637, -79.9182) (42.7499, -79.7375) (42.7353, -79.5572) (42.7198, -79.377) (42.7034, -79.1971) (42.6861, -79.0175) (42.6679, -78.8382) (42.6488, -78.6591) (42.6288, -78.4803) (42.6079, -78.3018) (42.586, -78.1236) (42.5631, -77.9457) (42.5394, -77.7681) (42.5146, -77.5908) (42.4889, -77.4138) (42.4622, -77.2372) (42.4345, -77.0609) (42.4058, -76.885) (42.376, -76.7094) (42.3451, -76.5342) (42.3133, -76.3593) (42.2803, -76.1848) (42.2464, -76.0108) (42.2113, -75.8371) (42.1752, -75.6638) (42.1379, -75.4909) (42.0993, -75.3185) (42.0595, -75.1467) (42.0184, -74.9753) (41.976, -74.8045) (41.9324, -74.6341) (41.8877, -74.4642) (41.8419, -74.2947) (41.7949, -74.1257) (41.7465, -73.9573) (41.6965, -73.7896) (41.6445, -73.6228) (41.5906, -73.4569) (41.5345, -73.2919) (41.4767, -73.1277) (41.4176, -72.9641) (41.3574, -72.801) (41.2964, -72.6383) (41.2339, -72.4763) (41.1689, -72.3156) (41.0997, -72.157) (41.0397, -72.0324) (40.9914, -71.9405) (40.9578, -71.88) (40.9406, -71.85) knots -1 -1 -1 -1 -1 -1 -0.98571429 -0.97142857 -0.95714286 -0.94285714 -0.92857143 -0.91428571 -0.9 -0.88571429 -0.87142857 -0.85714286 -0.84285714 -0.82857143 -0.81428571 -0.8 -0.78571429 -0.77142857 -0.75714286 -0.74285714 -0.72857143 -0.71428571 -0.7 -0.68571429 -0.67142857 -0.65714286 -0.64285714 -0.62857143 -0.61428571 -0.6 -0.58571429 -0.57142857 -0.55714286 -0.54285714 -0.52857143 -0.51428571 -0.5 -0.48571429 -0.47142857 -0.45714286 -0.44285714 -0.42857143 -0.41428571 -0.4 -0.38571429 -0.37142857 -0.35714286 -0.34285714 -0.32857143 -0.31428571 -0.3 -0.28571429 -0.27142857 -0.25714286 -0.24285714 -0.22857143 -0.21428571 -0.2 -0.18571429 -0.17142857 -0.15714286 -0.14285714 -0.12857143 -0.11428571 -0.1 -0.08571429 -0.07142857 -0.05714286 -0.04285714 -0.02857143 -0.01428571 0 0 0 0 0 0
  line L47 (40.9406, -71.85) -> (40.1986, -70.553)
  arc A95 (40.4866, -69.4737) -> (40.1986, -70.553) centre (40.8875, -70.1588) ccw
  arc A96 (40.4866, -69.4737) -> (44.8229, -66.7491) centre (-0.5538, 0.6546) ccw
  arc A97 (45.9202, -66.9578) -> (44.8229, -66.7491) centre (45.2661, -67.4076) ccw
  line L48 (45.9202, -66.9578) -> (46.7668, -68.1891)
  spline S48 degree 5 poles (46.7668, -68.1891) (46.7864, -68.2177) (46.8263, -68.2742) (46.8882, -68.3575) (46.9744, -68.4657) (47.0872, -68.5968) (47.2038, -68.7252) (47.3227, -68.8517) (47.4428, -68.9773) (47.5636, -69.1023) (47.6854, -69.2265) (47.8082, -69.3498) (47.9325, -69.4719) (48.0586, -69.5925) (48.1864, -69.7117) (48.3158, -69.8295) (48.4465, -69.9462) (48.5784, -70.0619) (48.7112, -70.1767) (48.8449, -70.2907) (48.9795, -70.4039) (49.115, -70.5162) (49.2516, -70.6276) (49.3891, -70.7381) (49.5277, -70.8476) (49.6672, -70.9562) (49.8077, -71.0639) (49.949, -71.1709) (50.0911, -71.277) (50.234, -71.3824) (50.3777, -71.487) (50.5222, -71.5908) (50.6674, -71.6938) (50.8135, -71.796) (50.9603, -71.8975) (51.1079, -71.9982) (51.2562, -72.0981) (51.4052, -72.1974) (51.5549, -72.2958) (51.7053, -72.3936) (51.8563, -72.4906) (52.0081, -72.587) (52.1604, -72.6826) (52.3135, -72.7775) (52.4672, -72.8717) (52.6215, -72.9652) (52.7765, -73.058) (52.932, -73.1501) (53.0882, -73.2416) (53.245, -73.3323) (53.4024, -73.4224) (53.5603, -73.5118) (53.7188, -73.6006) (53.878, -73.6887) (54.0376, -73.7761) (54.1978, -73.8629) (54.3586, -73.949) (54.5199, -74.0344) (54.6818, -74.1192) (54.8442, -74.2034) (55.0071, -74.2869) (55.1706, -74.3698) (55.3345, -74.452) (55.499, -74.5336) (55.664, -74.6146) (55.8295, -74.695) (55.9954, -74.7747) (56.1619, -74.8537) (56.3288, -74.9322) (56.4962, -75.01) (56.6641, -75.0873) (56.7988, -75.1485) (56.9001, -75.1942) (56.9677, -75.2245) (57.0015, -75.2397) knots 0 0 0 0 0 0 0.01428571 0.02857143 0.04285714 0.05714286 0.07142857 0.08571429 0.1 0.11428571 0.12857143 0.14285714 0.15714286 0.17142857 0.18571429 0.2 0.21428571 0.22857143 0.24285714 0.25714286 0.27142857 0.28571429 0.3 0.31428571 0.32857143 0.34285714 0.35714286 0.37142857 0.38571429 0.4 0.41428571 0.42857143 0.44285714 0.45714286 0.47142857 0.48571429 0.5 0.51428571 0.52857143 0.54285714 0.55714286 0.57142857 0.58571429 0.6 0.61428571 0.62857143 0.64285714 0.65714286 0.67142857 0.68571429 0.7 0.71428571 0.72857143 0.74285714 0.75714286 0.77142857 0.78571429 0.8 0.81428571 0.82857143 0.84285714 0.85714286 0.87142857 0.88571429 0.9 0.91428571 0.92857143 0.94285714 0.95714286 0.97142857 0.98571429 1 1 1 1 1 1
  arc A98 (57.0015, -75.2397) -> (60.6304, -72.3457) centre (-0.5538, 0.6546) ccw
  spline S49 degree 5 poles (60.6304, -72.3457) (60.6232, -72.3094) (60.6086, -72.2367) (60.5866, -72.1279) (60.5569, -71.9829) (60.5189, -71.8021) (60.4803, -71.6215) (60.441, -71.4413) (60.4009, -71.2614) (60.3601, -71.0819) (60.3186, -70.9027) (60.2764, -70.7238) (60.2334, -70.5453) (60.1897, -70.3672) (60.1453, -70.1894) (60.1001, -70.0119) (60.0542, -69.8349) (60.0075, -69.6582) (59.9601, -69.4819) (59.912, -69.306) (59.863, -69.1305) (59.8133, -68.9554) (59.7628, -68.7807) (59.7116, -68.6064) (59.6596, -68.4325) (59.6068, -68.259) (59.5532, -68.086) (59.4988, -67.9133) (59.4436, -67.7412) (59.3876, -67.5695) (59.3307, -67.3982) (59.2731, -67.2274) (59.2146, -67.0571) (59.1553, -66.8872) (59.0952, -66.7178) (59.0342, -66.549) (58.9723, -66.3806) (58.9096, -66.2127) (58.8461, -66.0454) (58.7816, -65.8786) (58.7163, -65.7123) (58.65, -65.5466) (58.5829, -65.3815) (58.5147, -65.2169) (58.4457, -65.053) (58.3757, -64.8896) (58.3048, -64.7268) (58.2329, -64.5647) (58.1601, -64.4031) (58.0863, -64.2422) (58.0115, -64.082) (57.9355, -63.9225) (57.8585, -63.7638) (57.7803, -63.6059) (57.7009, -63.4488) (57.6205, -63.2924) (57.5391, -63.1367) (57.4567, -62.9817) (57.3733, -62.8274) (57.2886, -62.6739) (57.2026, -62.5216) (57.1148, -62.3705) (57.0253, -62.2207) (56.9339, -62.0723) (56.841, -61.9251) (56.747, -61.7788) (56.6521, -61.6331) (56.5563, -61.4881) (56.4594, -61.3441) (56.3602, -61.2019) (56.2574, -61.0626) (56.1712, -60.9545) (56.1038, -60.8757) (56.0575, -60.8242) (56.034, -60.7988) knots -1 -1 -1 -1 -1 -1 -0.98571429 -0.97142857 -0.95714286 -0.94285714 -0.92857143 -0.91428571 -0.9 -0.88571429 -0.87142857 -0.85714286 -0.84285714 -0.82857143 -0.81428571 -0.8 -0.78571429 -0.77142857 -0.75714286 -0.74285714 -0.72857143 -0.71428571 -0.7 -0.68571429 -0.67142857 -0.65714286 -0.64285714 -0.62857143 -0.61428571 -0.6 -0.58571429 -0.57142857 -0.55714286 -0.54285714 -0.52857143 -0.51428571 -0.5 -0.48571429 -0.47142857 -0.45714286 -0.44285714 -0.42857143 -0.41428571 -0.4 -0.38571429 -0.37142857 -0.35714286 -0.34285714 -0.32857143 -0.31428571 -0.3 -0.28571429 -0.27142857 -0.25714286 -0.24285714 -0.22857143 -0.21428571 -0.2 -0.18571429 -0.17142857 -0.15714286 -0.14285714 -0.12857143 -0.11428571 -0.1 -0.08571429 -0.07142857 -0.05714286 -0.04285714 -0.02857143 -0.01428571 0 0 0 0 0 0
  line L49 (56.034, -60.7988) -> (55.022, -59.6994)
  arc A99 (55.0627, -58.5831) -> (55.022, -59.6994) centre (55.606, -59.1618) ccw
  arc A100 (55.0627, -58.5831) -> (58.6839, -54.9619) centre (-0.5538, 0.6546) ccw
  arc A101 (59.8002, -54.9212) -> (58.6839, -54.9619) centre (59.2626, -55.5052) ccw
  line L50 (59.8002, -54.9212) -> (60.8996, -55.9332)
  spline S50 degree 5 poles (60.8996, -55.9332) (60.925, -55.9567) (60.9765, -56.003) (61.0553, -56.0704) (61.1634, -56.1566) (61.3027, -56.2594) (61.4449, -56.3586) (61.5889, -56.4555) (61.7339, -56.5513) (61.8796, -56.6462) (62.0259, -56.7402) (62.1731, -56.8331) (62.3215, -56.9245) (62.4713, -57.014) (62.6224, -57.1018) (62.7747, -57.1878) (62.9282, -57.2725) (63.0824, -57.3559) (63.2375, -57.4383) (63.3932, -57.5197) (63.5496, -57.6001) (63.7067, -57.6795) (63.8646, -57.7577) (64.0233, -57.8347) (64.1828, -57.9107) (64.343, -57.9855) (64.5039, -58.0593) (64.6655, -58.1321) (64.8276, -58.204) (64.9904, -58.2749) (65.1538, -58.3449) (65.3177, -58.4139) (65.4823, -58.4821) (65.6474, -58.5492) (65.8131, -58.6155) (65.9794, -58.6808) (66.1462, -58.7453) (66.3135, -58.8088) (66.4814, -58.8715) (66.6498, -58.9334) (66.8186, -58.9944) (66.988, -59.0545) (67.1579, -59.1138) (67.3282, -59.1723) (67.499, -59.2299) (67.6703, -59.2868) (67.842, -59.3428) (68.0141, -59.398) (68.1868, -59.4524) (68.3598, -59.506) (68.5333, -59.5588) (68.7072, -59.6108) (68.8815, -59.662) (69.0562, -59.7125) (69.2313, -59.7622) (69.4068, -59.8112) (69.5827, -59.8593) (69.759, -59.9067) (69.9357, -59.9534) (70.1127, -59.9993) (70.2902, -60.0445) (70.468, -60.0889) (70.6461, -60.1326) (70.8246, -60.1756) (71.0035, -60.2178) (71.1827, -60.2593) (71.3622, -60.3001) (71.5421, -60.3402) (71.7223, -60.3795) (71.9029, -60.4181) (72.0837, -60.4561) (72.2287, -60.4858) (72.3375, -60.5078) (72.4102, -60.5224) (72.4465, -60.5296) knots 0 0 0 0 0 0 0.01428571 0.02857143 0.04285714 0.05714286 0.07142857 0.08571429 0.1 0.11428571 0.12857143 0.14285714 0.15714286 0.17142857 0.18571429 0.2 0.21428571 0.22857143 0.24285714 0.25714286 0.27142857 0.28571429 0.3 0.31428571 0.32857143 0.34285714 0.35714286 0.37142857 0.38571429 0.4 0.41428571 0.42857143 0.44285714 0.45714286 0.47142857 0.48571429 0.5 0.51428571 0.52857143 0.54285714 0.55714286 0.57142857 0.58571429 0.6 0.61428571 0.62857143 0.64285714 0.65714286 0.67142857 0.68571429 0.7 0.71428571 0.72857143 0.74285714 0.75714286 0.77142857 0.78571429 0.8 0.81428571 0.82857143 0.84285714 0.85714286 0.87142857 0.88571429 0.9 0.91428571 0.92857143 0.94285714 0.95714286 0.97142857 0.98571429 1 1 1 1 1 1
  arc A102 (72.4465, -60.5296) -> (75.3405, -56.9007) centre (-0.5538, 0.6546) ccw
  spline S51 degree 5 poles (75.3405, -56.9007) (75.3253, -56.8669) (75.295, -56.7993) (75.2493, -56.698) (75.1881, -56.5633) (75.1108, -56.3954) (75.033, -56.228) (74.9545, -56.0611) (74.8755, -55.8946) (74.7958, -55.7287) (74.7154, -55.5632) (74.6344, -55.3982) (74.5528, -55.2337) (74.4706, -55.0698) (74.3877, -54.9063) (74.3042, -54.7434) (74.22, -54.581) (74.1352, -54.4191) (74.0498, -54.2578) (73.9637, -54.097) (73.8769, -53.9368) (73.7895, -53.7772) (73.7014, -53.618) (73.6126, -53.4595) (73.5232, -53.3016) (73.4331, -53.1442) (73.3424, -52.9874) (73.2509, -52.8312) (73.1588, -52.6757) (73.066, -52.5207) (72.9725, -52.3664) (72.8783, -52.2127) (72.7834, -52.0596) (72.6878, -51.9073) (72.5914, -51.7555) (72.4944, -51.6045) (72.3966, -51.4541) (72.2982, -51.3044) (72.1989, -51.1554) (72.099, -51.0071) (71.9983, -50.8595) (71.8968, -50.7127) (71.7946, -50.5667) (71.6916, -50.4214) (71.5878, -50.2769) (71.4832, -50.1332) (71.3778, -49.9903) (71.2717, -49.8482) (71.1647, -49.7069) (71.057, -49.5664) (70.9484, -49.4269) (70.8389, -49.2883) (70.7284, -49.1508) (70.617, -49.0142) (70.5047, -48.8787) (70.3915, -48.7441) (70.2775, -48.6104) (70.1627, -48.4776) (70.047, -48.3457) (69.9303, -48.215) (69.8125, -48.0856) (69.6933, -47.9578) (69.5727, -47.8317) (69.4506, -47.7074) (69.3273, -47.5846) (69.2031, -47.4628) (69.0781, -47.342) (68.9525, -47.2219) (68.826, -47.103) (68.6976, -46.9865) (68.5664, -46.8736) (68.4583, -46.7874) (68.375, -46.7255) (68.3185, -46.6856) (68.2899, -46.666) knots -1 -1 -1 -1 -1 -1 -0.98571429 -0.97142857 -0.95714286 -0.94285714 -0.92857143 -0.91428571 -0.9 -0.88571429 -0.87142857 -0.85714286 -0.84285714 -0.82857143 -0.81428571 -0.8 -0.78571429 -0.77142857 -0.75714286 -0.74285714 -0.72857143 -0.71428571 -0.7 -0.68571429 -0.67142857 -0.65714286 -0.64285714 -0.62857143 -0.61428571 -0.6 -0.58571429 -0.57142857 -0.55714286 -0.54285714 -0.52857143 -0.51428571 -0.5 -0.48571429 -0.47142857 -0.45714286 -0.44285714 -0.42857143 -0.41428571 -0.4 -0.38571429 -0.37142857 -0.35714286 -0.34285714 -0.32857143 -0.31428571 -0.3 -0.28571429 -0.27142857 -0.25714286 -0.24285714 -0.22857143 -0.21428571 -0.2 -0.18571429 -0.17142857 -0.15714286 -0.14285714 -0.12857143 -0.11428571 -0.1 -0.08571429 -0.07142857 -0.05714286 -0.04285714 -0.02857143 -0.01428571 0 0 0 0 0 0
  line L51 (68.2899, -46.666) -> (67.0586, -45.8194)
  arc A103 (66.8499, -44.7221) -> (67.0586, -45.8194) centre (67.5084, -45.1653) ccw
  arc A104 (66.8499, -44.7221) -> (69.5745, -40.3858) centre (-0.5538, 0.6546) ccw
  arc A105 (70.6538, -40.0978) -> (69.5745, -40.3858) centre (70.2596, -40.7867) ccw
  line L52 (70.6538, -40.0978) -> (71.9508, -40.8398)
  spline S52 degree 5 poles (71.9508, -40.8398) (71.9808, -40.857) (72.0413, -40.8906) (72.1332, -40.9389) (72.2578, -40.9989) (72.4164, -41.0681) (72.5771, -41.1331) (72.7391, -41.1956) (72.9018, -41.2566) (73.0649, -41.3168) (73.2285, -41.3759) (73.3927, -41.4337) (73.5577, -41.4898) (73.7236, -41.5437) (73.8904, -41.5957) (74.0581, -41.6457) (74.2265, -41.6941) (74.3955, -41.7411) (74.565, -41.7869) (74.7349, -41.8316) (74.9053, -41.8752) (75.0761, -41.9176) (75.2475, -41.9587) (75.4193, -41.9985) (75.5917, -42.0371) (75.7646, -42.0744) (75.9378, -42.1105) (76.1116, -42.1456) (76.2856, -42.1795) (76.4601, -42.2125) (76.635, -42.2443) (76.8102, -42.2752) (76.9858, -42.305) (77.1617, -42.3337) (77.338, -42.3614) (77.5146, -42.3881) (77.6916, -42.4138) (77.8689, -42.4386) (78.0465, -42.4623) (78.2244, -42.4852) (78.4026, -42.5071) (78.5811, -42.528) (78.7599, -42.548) (78.939, -42.5671) (79.1183, -42.5853) (79.2979, -42.6026) (79.4778, -42.619) (79.658, -42.6345) (79.8383, -42.6491) (80.019, -42.6629) (80.1998, -42.6758) (80.381, -42.6878) (80.5623, -42.699) (80.7439, -42.7093) (80.9257, -42.7188) (81.1077, -42.7274) (81.2899, -42.7353) (81.4723, -42.7423) (81.6549, -42.7484) (81.8378, -42.7538) (82.0208, -42.7584) (82.204, -42.7621) (82.3874, -42.7651) (82.571, -42.7672) (82.7548, -42.7686) (82.9387, -42.7692) (83.1228, -42.769) (83.3071, -42.768) (83.4916, -42.7663) (83.6762, -42.7638) (83.861, -42.7605) (84.0089, -42.7573) (84.1199, -42.7545) (84.194, -42.7525) (84.231, -42.7515) knots 0 0 0 0 0 0 0.01428571 0.02857143 0.04285714 0.05714286 0.07142857 0.08571429 0.1 0.11428571 0.12857143 0.14285714 0.15714286 0.17142857 0.18571429 0.2 0.21428571 0.22857143 0.24285714 0.25714286 0.27142857 0.28571429 0.3 0.31428571 0.32857143 0.34285714 0.35714286 0.37142857 0.38571429 0.4 0.41428571 0.42857143 0.44285714 0.45714286 0.47142857 0.48571429 0.5 0.51428571 0.52857143 0.54285714 0.55714286 0.57142857 0.58571429 0.6 0.61428571 0.62857143 0.64285714 0.65714286 0.67142857 0.68571429 0.7 0.71428571 0.72857143 0.74285714 0.75714286 0.77142857 0.78571429 0.8 0.81428571 0.82857143 0.84285714 0.85714286 0.87142857 0.88571429 0.9 0.91428571 0.92857143 0.94285714 0.95714286 0.97142857 0.98571429 1 1 1 1 1 1
  arc A106 (84.231, -42.7515) -> (86.2449, -38.5696) centre (-0.5538, 0.6546) ccw